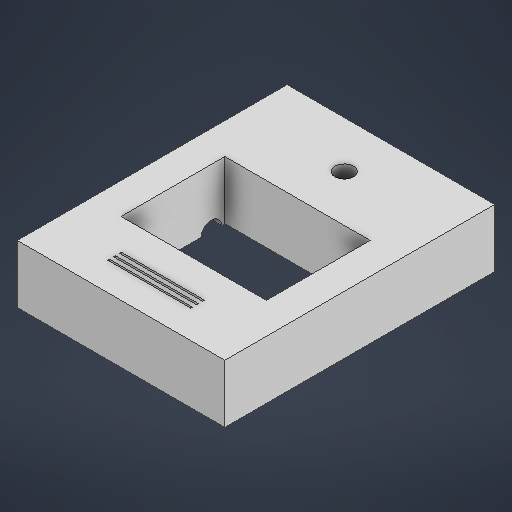
# Autodesk Inventor part: carcasaV2
Saved by Autodesk Inventor 2027.1 (Build 311270010, 270A)
## iProperties
Created: 2026-09-23
Part Number: carcasaV2
Material: Genérico
Document SubType Name: Sheet Metal
Designer: kadac
Density: 1 g/cm^3
Sheet Metal Rule: Por defecto_mm
Appearance: Valor por defecto
Author: kadac
Autodesk Inventor part; units mm, degrees
ref_plane "YZ Plane" through (0, 0, 0) normal (1, 0, 0) x (0, 1, 0)
ref_plane "XZ Plane" through (0, 0, 0) normal (0, 1, 0) x (-1, 0, 0)
ref_plane "XY Plane" through (0, 0, 0) normal (0, 0, 1) x (1, 0, 0)
sketch "Boceto1" plane through (0, 0, 0) normal (0, 1, 0) x (-1, 0, 0)
  line L0 (0, 0) -> (100, 0)
  line L1 (100, 0) -> (100, -130)
  line L2 (100, -130) -> (0, -130)
  line L3 (0, -130) -> (0, 0)
  dimension "d0" = 100
  dimension "d1" = 130
  constraints: 8 end point, 2 parallel, 1 horizontal, 1 perpendicular
  measures "d0" distance of L1.end L2.end
  measures "d1" distance of L0.end L1.end
extrude "Extrusión1" add sketch "Boceto1" along normal blind 28
sketch "Boceto2" plane through (0, 28, 0) normal (0, 1, 0) x (1, 0, 0)
  line L0 (-70, 13.56) -> (-30, 13.56)
  line L1 (-30, 13.56) -> (-30, 14.36)
  line L2 (-30, 14.36) -> (-70, 14.36)
  line L3 (-70, 14.36) -> (-70, 13.56)
  line L4 (-100, 0) -> (0, 0) projected
  line L5 (0, 0) -> (0, 130) projected
  line L6 (-70, 16.36) -> (-30, 16.36)
  line L7 (-30, 16.36) -> (-30, 17.26)
  line L8 (-30, 17.26) -> (-70, 17.26)
  line L9 (-70, 17.26) -> (-70, 16.36)
  line L10 (-70, 19.26) -> (-30, 19.26)
  line L11 (-30, 19.26) -> (-30, 20.16)
  line L12 (-30, 20.16) -> (-70, 20.16)
  line L13 (-70, 20.16) -> (-70, 19.26)
  line L14 (-85, 85) -> (-15, 85)
  line L15 (-15, 85) -> (-15, 35)
  line L16 (-15, 35) -> (-85, 35)
  line L17 (-85, 35) -> (-85, 85)
  line L18 (-100, 130) -> (-100, 0) projected
  line L19 (0, 130) -> (-100, 130) projected
  circle A0 centre (-50, 107.5) radius 4.5
  dimension "d4" = 40
  dimension "d5" = 0.8
  dimension "d6" = 13.56
  dimension "d7" = 30
  dimension "d8" = 40
  dimension "d9" = 0.9
  dimension "d10" = 2
  dimension "d11" = 0
  dimension "d12" = 40
  dimension "d13" = 0.9
  dimension "d14" = 0
  dimension "d15" = 2
  dimension "d16" = 70
  dimension "d17" = 50
  dimension "d18" = 15
  dimension "d19" = 45
  dimension "d20" = 9
  dimension "d21" = 50
  dimension "d22" = 22.5
  constraints: 32 end point, 8 parallel, 4 horizontal, 4 perpendicular, 1 centre point
  measures "d4" distance of L2.end L1.end
  measures "d5" distance of L1.end L0.end
  measures "d6" distance from line of L4 L0.end
  measures "d7" distance from line of L5 L0.end
  measures "d8" distance of L8.end L7.end
  measures "d9" distance of L7.end L6.end
  measures "d10" distance between parallel lines of L2 L6
  measures "d11" distance between parallel lines of L7 L1
  measures "d12" distance of L12.end L11.end
  measures "d13" distance of L11.end L10.end
  measures "d14" distance between parallel lines of L11 L7
  measures "d15" distance between parallel lines of L8 L10
  measures "d16" distance of L15.end L16.end
  measures "d17" distance of L14.end L15.end
  measures "d18" distance between parallel lines of L18 L17
  measures "d19" distance between parallel lines of L19 L14
  measures "d20" diameter of A0
  measures "d21" distance from line of L5 A0.centre
  measures "d22" distance from line of L19 A0.centre
extrude "Extrusión2" cut sketch "Boceto2" against normal blind 28 contours L3 L2 L1 L0 | L9 L8 L7 L6 | L13 L12 L11 L10 | L14 L15 L16 L17 | A0
sketch "Boceto3" plane through (-100, 0, -130) normal (-1, 0, 0) x (0, 0, 1)
  line L0 (95, 0) -> (45, 0) projected
  arc A0 (56.5512, 0) -> (46.5113, 0) centre (51.5312, -0.2684) ccw
  point P0 (130, 0)
  constraints: 2 point on circle, 2 point on line, 1 centre point
extrude "Extrusión3" cut sketch "Boceto3" against normal blind 15
equation "\"Radio_pliegue\" = Grosor"
equation "\"Anchura_desahogo_plegado\" = Grosor"
equation "\"Profundidad_desahogo_plegado\" = 0.5 * Grosor"
equation "\"Tamaño_destalonado\" = 4 * Grosor"
equation "\"Remanente_mínimo\" = 2 * Grosor"
equation "\"Radiodetransición\" = Radio_pliegue"
equation "\"Tamaño_de_radio_de_Jacobi\" = Radio_pliegue"
equation "\"TamañoSeparación\" = Grosor"
equation "\"Grosor\" = 0.5"
